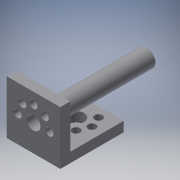
# Autodesk Inventor part: Flag Mount
Saved by Autodesk Inventor 2016 (Build 200138000, 138)
## iProperties
Created: 2016-01-18
Part Number: Flag Mount
Material: Generic
Document SubType Name: Modeling
Designer: tbloo
Density: 1 g/cm^3
Appearance: Default
Author: tbloo
Autodesk Inventor part; units mm, degrees
ref_plane "YZ Plane" through (0, 0, 0) normal (1, 0, 0) x (0, 1, 0)
ref_plane "XZ Plane" through (0, 0, 0) normal (0, 1, 0) x (-1, 0, 0)
ref_plane "XY Plane" through (0, 0, 0) normal (0, 0, 1) x (1, 0, 0)
sketch "Sketch1" plane through (0, 0, 0) normal (0, 1, 0) x (-1, 0, 0)
  line L0 (-13.5, -13.5) -> (13.5, -13.5)
  line L1 (13.5, -13.5) -> (13.5, 13.5)
  line L2 (13.5, 13.5) -> (-13.5, 13.5)
  line L3 (-13.5, 13.5) -> (-13.5, -13.5)
  line L4 (-13.5, -13.5) -> (13.5, 13.5) construction
  line L5 (13.5, -13.5) -> (-13.5, 13.5) construction
  circle A0 centre (0, 0) radius 3.5
  dimension "d0" = 27
  dimension "d1" = 27
  dimension "d5" = 7
  constraints: 12 end point, 2 midpoint, 2 parallel, 1 centre point, 1 coincident, 1 horizontal, 1 perpendicular
  measures "d0" distance of L2.end L1.end
  measures "d1" distance of L1.end L0.end
  measures "d5" diameter of A0
extrude "Extrusion2" add sketch "Sketch1" along normal blind 5
sketch "Sketch4" plane through (0, 5, 0) normal (0, 1, 0) x (1, 0, 0)
  line L0 (-13.5, 13.5) -> (-13.5, -13.5) projected
  line L1 (-13.5, 13.5) -> (13.5, 13.5)
  line L2 (13.5, 13.5) -> (13.5, 8.5)
  line L3 (13.5, 8.5) -> (-13.5, 8.5)
  line L4 (-13.5, 8.5) -> (-13.5, 13.5)
  point P0 (0, 0)
  dimension "d11" = 27
  dimension "d12" = 5
  constraints: 8 end point, 2 parallel, 1 horizontal, 1 perpendicular
  measures "d11" distance of L2.end L3.end
  measures "d12" distance of L1.end L2.end
extrude "Extrusion4" add sketch "Sketch4" along normal blind 27
sketch "Sketch5" plane through (13.5, 0, -13.5) normal (0, 0, -1) x (-1, 0, 0)
  line L0 (27, 5) -> (27, 32) projected
  line L1 (0, 32) -> (27, 32)
  line L2 (27, 32) -> (27, 5)
  line L3 (27, 5) -> (0, 5)
  line L4 (0, 5) -> (0, 32)
  circle A0 centre (13.5, 21.5) radius 4
  point P0 (13.5, 0)
  dimension "d15" = 27
  dimension "d16" = 27
  dimension "d17" = 8
  constraints: 8 end point, 2 parallel, 1 centre point, 1 horizontal, 1 perpendicular
  measures "d15" distance of L0.start L3.end
  measures "d16" distance of L1.end L0.start
  measures "d17" diameter of A0
hole "Hole1" at (0, 21.5, -13.5) direction (0, 0, 1) diameter 8 depth 5 tip angle 118
sketch "Sketch7" plane through (0, 0, 0) normal (0, -1, 0) x (1, 0, 0)
  circle A0 centre (8, 0) radius 1.85 projected
  circle A1 centre (5.6569, 5.6569) radius 1.85 projected
  circle A2 centre (0, 8) radius 1.85 projected
  circle A3 centre (-5.6569, 5.6569) radius 1.85 projected
  circle A4 centre (-8, 0) radius 1.85 projected
  point P0 (0, 0)
hole "Hole2" at (8, 0, 0) at (5.6569, 0, 5.6569) at (0, 0, 8) at (-5.6569, 0, 5.6569) at (-8, 0, 0) direction (0, 1, 0) diameter 4 end through all
sketch "Sketch9" plane through (0, 5, 0) normal (0, 1, 0) x (1, 0, 0)
  circle A0 centre (0, 0) radius 4.5
  circle A1 centre (0, 0) radius 3.5 projected
  dimension "d33" = 9
  constraints: 1 centre point, 1 coincident
  measures "d33" diameter of A0
extrude "Extrusion5" add sketch "Sketch9" along normal blind 52
sketch "Sketch10" plane through (13.5, 0, -13.5) normal (0, 0, -1) x (-1, 0, 0)
  circle A0 centre (21.5, 21.5) radius 1.85
  circle A1 centre (5.5, 21.5) radius 1.85
  circle A2 centre (19.1569, 27.1569) radius 1.85
  circle A3 centre (19.1569, 15.8431) radius 1.85
  circle A4 centre (7.8431, 15.8431) radius 1.85
  circle A5 centre (7.8431, 27.1569) radius 1.85
  point P0 (13.5, 0)
  constraints: 6 centre point, 12 other
hole "Hole3" at (5.6569, 15.8431, -13.5) at (8, 21.5, -13.5) at (5.6569, 27.1569, -13.5) at (-5.6569, 27.1569, -13.5) at (-8, 21.5, -13.5) at (-5.6569, 15.8431, -13.5) direction (0, 0, 1) diameter 4 depth 5 tip angle 118
body "Solid2"
